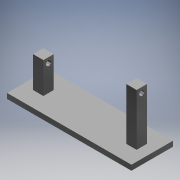
# Autodesk Inventor part: base
Saved by Autodesk Inventor 2019 Beta2 (Build 230110000, 110) ContinuousBuild 0
## iProperties
Created: 2014-03-04
Part Number: base
Material: Silicon Nitride
Document SubType Name: Modeling
Designer: John
Density: 3.18 g/cm^3
Appearance: Chrome - Polished Black
Mass: 205.885 g
Surface Area: 236.058 cm^2
Volume: 64.7439 cm^3
Author: John
Autodesk Inventor part; units mm, degrees
ref_plane "YZ Plane" through (0, 0, 0) normal (1, 0, 0) x (0, 1, 0)
ref_plane "XZ Plane" through (0, 0, 0) normal (0, 1, 0) x (-1, 0, 0)
ref_plane "XY Plane" through (0, 0, 0) normal (0, 0, 1) x (1, 0, 0)
sketch "Sketch1" plane through (0, 0, 0) normal (0, 0, 1) x (1, 0, 0)
  line L0 (-76.2, -25.4) -> (76.2, -25.4)
  line L1 (76.2, -25.4) -> (76.2, 25.4)
  line L2 (76.2, 25.4) -> (-76.2, 25.4)
  line L3 (-76.2, 25.4) -> (-76.2, -25.4)
  line L4 (-76.2, -25.4) -> (76.2, 25.4) construction
  line L5 (76.2, -25.4) -> (-76.2, 25.4) construction
  point P0 (0, 0)
  dimension "d0" = 152.4
  dimension "d1" = 50.8
  constraints: 12 end point, 2 midpoint, 2 parallel, 1 horizontal, 1 perpendicular
  measures "d0" distance of L2.end L1.end
  measures "d1" distance of L1.end L0.end
extrude "Extrusion1" add sketch "Sketch1" along normal blind 6.35
sketch "Sketch2" plane through (0, 0, 6.35) normal (0, 0, 1) x (1, 0, 0)
  line L0 (-76.2, 25.4) -> (-76.2, -25.4) projected
  line L1 (-63.5, 6.35) -> (-50.8, 6.35)
  line L2 (-50.8, 6.35) -> (-50.8, -6.35)
  line L3 (-50.8, -6.35) -> (-63.5, -6.35)
  line L4 (-63.5, -6.35) -> (-63.5, 6.35)
  point P0 (0, 0)
  dimension "d4" = 12.7
  dimension "d5" = 12.7
  dimension "d6" = 6.35
  dimension "d7" = 12.7
  constraints: 8 end point, 2 parallel, 1 horizontal, 1 perpendicular
  measures "d4" distance of L3.end L1.start
  measures "d5" distance of L1.start L1.end
  measures "d6" distance from line of point (0, 0) L1
  measures "d7" distance between parallel lines of L0 L4
extrude "Extrusion2" add sketch "Sketch2" along normal blind 38.1
sketch "Sketch3" plane through (0, 0, 6.35) normal (0, 0, 1) x (1, 0, 0)
  line L0 (76.2, -25.4) -> (76.2, 25.4) projected
  line L1 (50.8, -6.35) -> (63.5, -6.35)
  line L2 (63.5, -6.35) -> (63.5, 6.35)
  line L3 (63.5, 6.35) -> (50.8, 6.35)
  line L4 (50.8, 6.35) -> (50.8, -6.35)
  point P0 (0, 0)
  dimension "d10" = 12.7
  dimension "d11" = 12.7
  dimension "d12" = 6.35
  dimension "d13" = 12.7
  constraints: 8 end point, 2 parallel, 1 horizontal, 1 perpendicular
  measures "d10" distance of L2.end L3.end
  measures "d11" distance of L3.end L1.start
  measures "d12" distance from line of point (0, 0) L3
  measures "d13" distance between parallel lines of L0 L2
extrude "Extrusion3" add sketch "Sketch3" along normal blind 63.5
sketch "Sketch4" plane through (63.5, -6.35, 6.35) normal (1, 0, 0) x (0, 0, -1)
  circle A0 centre (-57.15, 6.35) radius 3.175
  line L0 (0, 12.7) -> (-63.5, 12.7) projected
  line L1 (-63.5, 0) -> (-63.5, 12.7) projected
  point P0 (6.35, 6.35)
  dimension "d16" = 6.35
  dimension "d19" = 6.35
  dimension "d20" = 6.35
  constraints: 1 centre point
  measures "d16" diameter of A0
  measures "d19" distance from line of L1 A0.centre
  measures "d20" distance from line of L0 A0.centre
extrude "Extrusion4" cut sketch "Sketch4" against normal through all
sketch "Sketch5" plane through (-50.8, -6.35, 6.35) normal (1, 0, 0) x (0, 0, -1)
  line L0 (0, 12.7) -> (-38.1, 12.7) projected
  line L1 (-38.1, 0) -> (-38.1, 12.7) projected
  circle A0 centre (-31.75, 6.35) radius 3.175
  point P0 (6.35, 6.35)
  dimension "d21" = 6.35
  dimension "d22" = 6.35
  dimension "d23" = 6.35
  constraints: 1 centre point
  measures "d21" diameter of A0
  measures "d22" distance from line of L0 A0.centre
  measures "d23" distance from line of L1 A0.centre
extrude "Extrusion5" cut sketch "Sketch5" against normal through all
equation "\"d5\" = d4"
equation "\"d6\" = 0.5 * d4"
equation "\"d12\" = 0.5 * d11"
body "Solid1"
